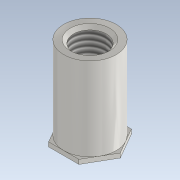
# Autodesk Inventor part: Вытяжная заклепка_Р-Ш-М3-Ум
Saved by Autodesk Inventor 2021.2 (Build 252289000, 289)
## iProperties
Created: 2009-05-22
Part Number: Вытяжная заклепка_Р-Ш-М3-Ум
Document SubType Name: Modeling
Designer: svb
Density: 7.85 g/cm^3
Material: Сталь низкоуглеродистая
Mass: 0.789415 g
Surface Area: 2.50949 cm^2
Volume: 0.100562 cm^3
Appearance: Сталь
Author: svb
Autodesk Inventor part; units mm, degrees
ref_plane "YZ Plane" through (0, 0, 0) normal (1, 0, 0) x (0, 1, 0)
ref_plane "XZ Plane" through (0, 0, 0) normal (0, 1, 0) x (-1, 0, 0)
ref_plane "XY Plane" through (0, 0, 0) normal (0, 0, 1) x (1, 0, 0)
sketch "Sketch1" plane through (0, 0, 0) normal (0, 0, 1) x (1, 0, 0)
  line L0 (1.4722, 2.55) -> (2.9445, 0)
  line L1 (2.9445, 0) -> (1.4722, -2.55)
  line L2 (1.4722, -2.55) -> (-1.4722, -2.55)
  line L3 (-1.4722, -2.55) -> (-2.9445, 0)
  line L4 (-2.9445, 0) -> (-1.4722, 2.55)
  line L5 (-1.4722, 2.55) -> (1.4722, 2.55)
  point P0 (0, 0)
  dimension "d0" = 5.1
  constraints: 12 end point, 13 other
  measures "d0" distance between parallel lines of L2 L5
extrude "Extrusion1" add sketch "Sketch1" along normal blind 0.4
sketch "Sketch2" plane through (0, 0, 0.4) normal (0, 0, 1) x (1, 0, 0)
  circle A0 centre (0, 0) radius 2.4
  dimension "d3" = 4.8
  constraints: 1 centre point
  measures "d3" diameter of A0
extrude "Extrusion2" add sketch "Sketch2" along normal blind 8.6
sketch "Sketch3" plane through (0, 0, 9) normal (0, 0, 1) x (1, 0, 0)
  circle A0 centre (0, 0) radius 2.4 projected
  circle A1 centre (0, 0) radius 1.5
  dimension "d6" = 3
  constraints: 1 centre point, 1 coincident
  measures "d6" diameter of A1
extrude "Extrusion3" cut sketch "Sketch3" against normal blind 10 contours A1
chamfer "Chamfer1" distance 0.3 angle 45 1 edges at (-1.5, 0, 9)
thread "Thread1" size "M3x0.5" class "6H" standard "ANSI Metric M Profile" full length
